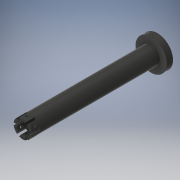
# Autodesk Inventor part: TA03
Saved by Autodesk Inventor 2017 (Build 210142000, 142)
## iProperties
Created: 2018-10-09
Part Number: TA03
Material: ABS Plastic
Document SubType Name: Modeling
Designer: Zach
Density: 1.06 g/cm^3
Appearance: Smooth - Black
Author: Zach
Autodesk Inventor part; units mm, degrees
ref_plane "YZ Plane" through (0, 0, 0) normal (1, 0, 0) x (0, 1, 0)
ref_plane "XZ Plane" through (0, 0, 0) normal (0, 1, 0) x (-1, 0, 0)
ref_plane "XY Plane" through (0, 0, 0) normal (0, 0, 1) x (1, 0, 0)
sketch "Sketch1" plane through (0, 0, 0) normal (0, 0, 1) x (1, 0, 0)
  circle A0 centre (0, 0) radius 7.5
  circle A1 centre (0, 0) radius 10
  dimension "d0" = 15
  dimension "d1" = 20
  constraints: 2 centre point, 2 coincident
  measures "d0" diameter of A0
  measures "d1" diameter of A1
extrude "Extrusion1" add sketch "Sketch1" along normal blind 145
sketch "Sketch2" plane through (0, 0, 0) normal (0, 0, -1) x (-1, 0, 0)
  circle A0 centre (0, 0) radius 17.5
  circle A1 centre (0, 0) radius 7.5 projected
  dimension "d4" = 35
  constraints: 1 centre point, 1 coincident
  measures "d4" diameter of A0
extrude "Extrusion2" add sketch "Sketch2" along normal blind 7
sketch "Sketch4" plane through (0, 0, 145) normal (0, 0, 1) x (1, 0, 0)
  line L0 (0, 1.5) -> (10, 1.5)
  line L1 (10, 1.5) -> (10, -1.5)
  line L2 (10, -1.5) -> (0, -1.5)
  line L3 (0, -1.5) -> (0, 1.5)
  circle A0 centre (0, 0) radius 10 construction
  line L4 (-1.299, 0.75) -> (3.701, 9.4103)
  line L5 (3.701, 9.4103) -> (6.299, 7.9103)
  line L6 (6.299, 7.9103) -> (1.299, -0.75)
  line L7 (1.299, -0.75) -> (-1.299, 0.75)
  line L8 (-1.299, -0.75) -> (-6.299, 7.9103)
  line L9 (-6.299, 7.9103) -> (-3.701, 9.4103)
  line L10 (-3.701, 9.4103) -> (1.299, 0.75)
  line L11 (1.299, 0.75) -> (-1.299, -0.75)
  line L12 (0, -1.5) -> (-10, -1.5)
  line L13 (-10, -1.5) -> (-10, 1.5)
  line L14 (-10, 1.5) -> (0, 1.5)
  line L15 (0, 1.5) -> (0, -1.5)
  line L16 (1.299, -0.75) -> (-3.701, -9.4103)
  line L17 (-3.701, -9.4103) -> (-6.299, -7.9103)
  line L18 (-6.299, -7.9103) -> (-1.299, 0.75)
  line L19 (-1.299, 0.75) -> (1.299, -0.75)
  line L20 (1.299, 0.75) -> (6.299, -7.9103)
  line L21 (6.299, -7.9103) -> (3.701, -9.4103)
  line L22 (3.701, -9.4103) -> (-1.299, -0.75)
  line L23 (-1.299, -0.75) -> (1.299, 0.75)
  point P0 (10, 0)
  point P1 (5, 8.6603)
  point P2 (-5, 8.6603)
  point P3 (-10, 0)
  point P4 (-5, -8.6603)
  point P5 (5, -8.6603)
  dimension "d14" = 3
  dimension "d17" = 360
  constraints: 48 end point, 8 coincident, 2 midpoint, 2 parallel, 1 horizontal, 1 horizontal alignment, 1 perpendicular, 72 other
  measures "d14" distance of L2.end L0.start
extrude "Extrusion4" cut sketch "Sketch4" against normal blind 10
sketch "Sketch8" plane through (0, 0, 0) normal (0, 1, 0) x (-1, 0, 0)
  line L0 (3.6444, 145) -> (-3.6444, 145) projected
  line L1 (3.6444, 135) -> (3.6444, 145) projected
  circle A0 centre (0, 140) radius 1.5
  point P0 (0, 0)
  point P1 (0, 145)
  point P2 (3.6444, 140)
  dimension "d21" = 3
  constraints: 2 midpoint, 1 centre point, 1 horizontal alignment, 1 vertical alignment
  measures "d21" diameter of A0
extrude "Extrusion5" cut sketch "Sketch8" along normal through all both and the other way through all
pattern_circular "Circular Pattern1" count 6 over 360 about axis through (0, 0, -10) along (0, 0, 1) of "Extrusion5"
body "Solid1"
